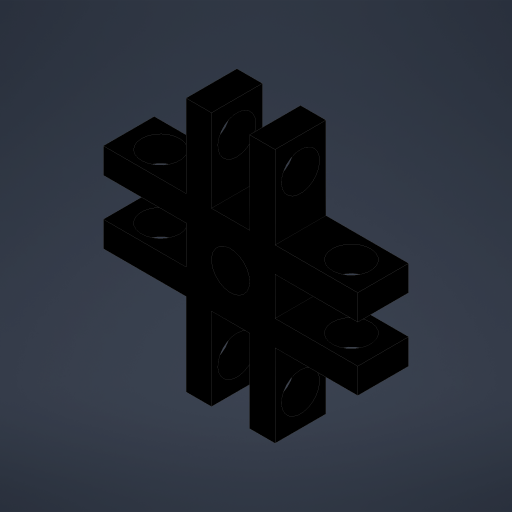
# Autodesk Inventor part: Center Connector
Saved by Autodesk Inventor 2023 (Build 270158000, 158)
## iProperties
Created: 2023-04-12
Part Number: Center Connector
Material: Generic
Document SubType Name: Modeling
Designer: vatdu
Density: 1 g/cm^3
Appearance: Default
Author: vatdu
Autodesk Inventor part; units mm, degrees
ref_plane "YZ Plane" through (0, 0, 0) normal (1, 0, 0) x (0, 1, 0)
ref_plane "XZ Plane" through (0, 0, 0) normal (0, 1, 0) x (-1, 0, 0)
ref_plane "XY Plane" through (0, 0, 0) normal (0, 0, 1) x (1, 0, 0)
sketch "Sketch1" plane through (0, 0, 0) normal (0, 0, 1) x (1, 0, 0)
  line L0 (0, 0) -> (20, 0)
  line L1 (20, 0) -> (20, 20)
  line L2 (20, 20) -> (0, 20)
  line L3 (0, 20) -> (0, 0)
  line L4 (8.4977, 20) -> (6.4977, 20)
  line L5 (6.4977, 0) -> (8.4977, 0)
  line L6 (0, 3.9) -> (0, 5.9)
  line L7 (20, 8.9) -> (20, 10.9)
  line L8 (0, 10.9) -> (0, 8.9)
  line L9 (10, 0) -> (10, 10)
  circle A0 centre (10, 10) radius 1.5
  line L10 (0, 11.5) -> (20, 11.5)
  line L11 (20, 11.5) -> (20, 13.5)
  line L12 (20, 13.5) -> (0, 13.5)
  line L13 (0, 13.5) -> (0, 11.5)
  line L14 (6.5, 20) -> (6.5, 0)
  line L15 (8.5, 0) -> (8.5, 20)
  line L16 (0, 6.5) -> (20, 6.5)
  line L17 (20, 8.5) -> (0, 8.5)
  line L18 (13.5, 0) -> (13.5, 20)
  line L19 (11.5, 20) -> (11.5, 0)
  point P0 (6.5, 11.5)
  point P1 (6.5, 8.5)
  point P2 (6.5, 6.5)
  point P3 (6.5, 0)
  point P4 (8.5, 6.5)
  point P5 (10, 6.5)
  point P6 (13.5, 6.5)
  point P7 (13.5, 8.5)
  point P8 (13.5, 11.5)
  point P9 (13.5, 13.5)
  point P10 (11.5, 13.5)
  point P11 (8.5, 13.5)
  point P12 (6.5, 13.5)
  point P13 (0, 13.5)
  point P14 (11.5, 6.5)
  dimension "d0" = 20
  dimension "d1" = 20
  dimension "d7" = 2
  dimension "d10" = 2
  dimension "d19" = 10
  dimension "d20" = 3
  dimension "d21" = 20
  dimension "d22" = 2
  dimension "d25" = 360
  constraints: 40 end point, 6 parallel, 6 point on line, 3 horizontal, 2 perpendicular, 1 centre point, 1 coincident, 1 midpoint, 1 vertical, 25 other
  measures "d0" distance of L2.end L1.end
  measures "d1" distance of L1.end L0.end
  measures "d7" distance of L5.end L5.start
  measures "d10" distance of L7.end L7.start
  measures "d19" distance of L9.start L9.end
  measures "d20" diameter of A0
  measures "d21" distance of L12.end L11.end
  measures "d22" distance of L11.end L10.end
extrude "Extrusion1" add sketch "Sketch1" along normal blind 4 contours L14 L16 L15 L0 | L16 L3 L17 L14 | L14 L17 L15 L16 | L14 L10 L15 L17 | L15 L17 L9 L16 | L14 L12 L15 L10 | L10 L3 L12 L14 | L15 A0 L17 | L9 L17 L19 L16 | L19 L16 L18 L0 | L15 L12 L19 L10 | L10 A0 L15 | L14 L2 L15 L12 | A0 L19 L17 | L19 L17 L18 L16 | L10 L19 A0 | L19 L10 L18 L17 | L18 L17 L1 L16 | L19 L12 L18 L10 | L19 L2 L18 L12 | L18 L12 L1 L10
sketch "Sketch3" plane through (13.5, 6.5, 0) normal (0, -1, 0) x (1, 0, 0)
  line L0 (0, 0) -> (0, 4) projected
  line L1 (0, 0) -> (4, 0)
  line L2 (0, 0) -> (6.5, 0) projected
  line L3 (4, 0) -> (4, 2)
  circle A0 centre (4, 2) radius 1.5
  point P0 (-13.5, 0)
  dimension "d27" = 4
  dimension "d28" = 2
  dimension "d29" = 3
  constraints: 4 end point, 1 centre point, 1 coincident, 1 perpendicular, 1 point on line
  measures "d27" distance of L0.start L1.end
  measures "d28" distance of L1.end L3.end
  measures "d29" diameter of A0
extrude "Extrusion3" cut sketch "Sketch3" against normal blind 10
pattern_circular "Circular Pattern2" count 4 over 360 about axis through (10, 10, 0) along (0, 0, 1) of "Extrusion3"
body "Solid1"
